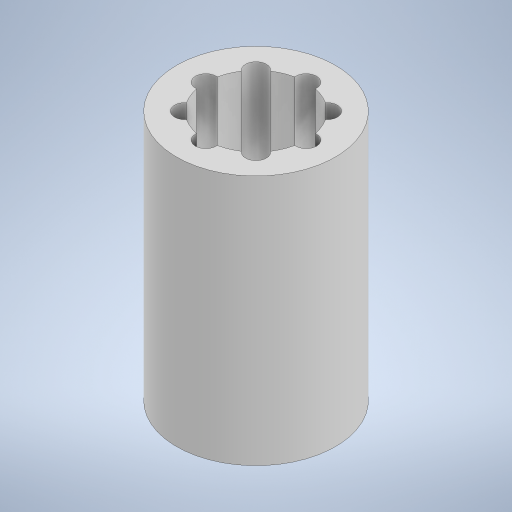
# Autodesk Inventor part: Bearing
Saved by Autodesk Inventor 2023 (Build 270158000, 158)
## iProperties
Created: 2023-04-11
Part Number: Bearing
Material: Generic
Document SubType Name: Modeling
Designer: Nathann
Density: 1 g/cm^3
Appearance: Default
Author: Nathann
Autodesk Inventor part; units mm, degrees
ref_plane "YZ Plane" through (0, 0, 0) normal (1, 0, 0) x (0, 1, 0)
ref_plane "XZ Plane" through (0, 0, 0) normal (0, 1, 0) x (-1, 0, 0)
ref_plane "XY Plane" through (0, 0, 0) normal (0, 0, 1) x (1, 0, 0)
sketch "Sketch1" plane through (0, 0, 0) normal (0, 1, 0) x (-1, 0, 0)
  circle A0 centre (0, 0) radius 6
  circle A1 centre (0, 0) radius 9.5
  circle A2 centre (6, 0) radius 1.25
  line L0 (6, 0) -> (4.0311, 0)
  circle A3 centre (4.2426, 4.2426) radius 1.25
  circle A4 centre (0, 6) radius 1.25
  circle A5 centre (-4.2426, 4.2426) radius 1.25
  circle A6 centre (-6, 0) radius 1.25
  circle A7 centre (-4.2426, -4.2426) radius 1.25
  circle A8 centre (0, -6) radius 1.25
  circle A9 centre (4.2426, -4.2426) radius 1.25
  point P0 (5.8698, -1.2432)
  point P1 (5.8698, 1.2432)
  point P2 (5.0296, -3.2715)
  point P3 (3.2715, -5.0296)
  point P4 (1.2432, -5.8698)
  point P5 (-1.2432, -5.8698)
  point P6 (-3.2715, -5.0296)
  point P7 (-5.0296, -3.2715)
  point P8 (-5.8698, -1.2432)
  point P9 (-5.8698, 1.2432)
  point P10 (-5.0296, 3.2715)
  point P11 (-3.2715, 5.0296)
  point P12 (-1.2432, 5.8698)
  point P13 (1.2432, 5.8698)
  point P14 (3.2715, 5.0296)
  point P15 (5.0296, 3.2715)
  dimension "d1" = 12
  dimension "d0" = 19
  dimension "d2" = 2.5
  dimension "d14" = 6
  dimension "d15" = 2.25
  dimension "d18" = 360
  dimension "d20" = 4.2426
  dimension "d21" = 4.2426
  dimension "d22" = 6
  constraints: 9 centre point, 2 coincident, 2 end point, 1 horizontal, 20 other
  measures "d0" diameter of A1
  measures "d2" diameter of A2
  measures "d14" distance of point (0, 0) L0.start
  measures "d20" horizontal distance of point (0, 0) A7.centre
  measures "d21" horizontal distance of point (0, 0) A7.centre
  measures "d22" distance of point (0, 0) A6.centre
extrude "Extrusion1" add sketch "Sketch1" along normal blind 30
body "Solid1"
